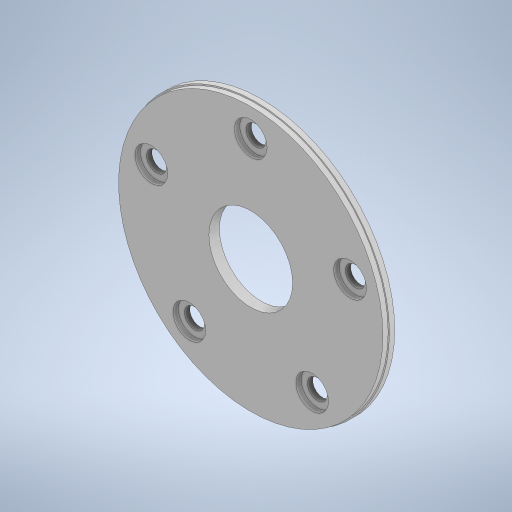
# Autodesk Inventor part: Savior Paddle Template
Saved by Autodesk Inventor 2024 (Build 280153000, 153)
## iProperties
Created: 2023-12-08
Part Number: Savior Paddle Template
Material: Generic
Document SubType Name: Modeling
Designer: luke.macenski3281
Density: 1 g/cm^3
Appearance: Default
Author: luke.macenski3281
Autodesk Inventor part; units mm, degrees
ref_plane "YZ Plane" through (0, 0, 0) normal (1, 0, 0) x (0, 1, 0)
ref_plane "XZ Plane" through (0, 0, 0) normal (0, 1, 0) x (-1, 0, 0)
ref_plane "XY Plane" through (0, 0, 0) normal (0, 0, 1) x (1, 0, 0)
sketch "Sketch1" plane through (0, 0, 0) normal (0, 0, 1) x (1, 0, 0)
  circle A0 centre (0, 0) radius 20.32
  circle A1 centre (0, 0) radius 64.77
  circle A2 centre (0, 50.7238) radius 4.8601
  circle A3 centre (-48.2412, 15.6745) radius 4.8601
  circle A4 centre (-29.8147, -41.0364) radius 4.8601
  circle A5 centre (29.8147, -41.0364) radius 4.8601
  circle A6 centre (48.2412, 15.6745) radius 4.8601
  dimension "d0" = 40.64
  dimension "d1" = 129.54
  dimension "d2" = 50.7238
  dimension "d5" = 360
  constraints: 7 centre point, 2 coincident, 11 other
  measures "d0" diameter of A0
  measures "d1" diameter of A1
  measures "d2" distance of point (0, 0) A2.centre
extrude "Extrusion1" add sketch "Sketch1" along normal blind 2.54
sketch "Sketch2" plane through (0, 0, 2.54) normal (0, 0, 1) x (1, 0, 0)
  circle A0 centre (0, 0) radius 20.32 projected
  circle A1 centre (0, 0) radius 20.32
  circle A2 centre (0, 0) radius 64.1368
  circle A3 centre (0, 50.7238) radius 4.8601 projected
  circle A4 centre (0, 50.7238) radius 7.9502
  circle A5 centre (-48.2412, 15.6745) radius 7.9502
  circle A6 centre (-29.8147, -41.0364) radius 7.9502
  circle A7 centre (29.8147, -41.0364) radius 7.9502
  circle A8 centre (48.2412, 15.6745) radius 7.9502
  dimension "d9" = 15.9004
  dimension "d12" = 360
  constraints: 7 centre point, 5 coincident, 14 other
  measures "d9" diameter of A4
extrude "Extrusion2" add sketch "Sketch2" along normal blind 2.54 contours A2
body "Solid1"
